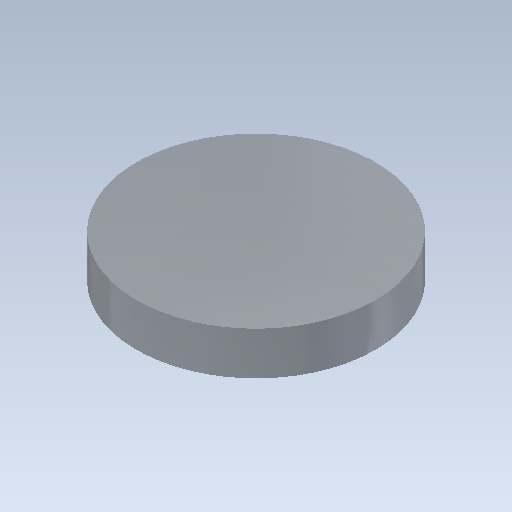
# Autodesk Inventor part: Borosilikatglas 55x10
Saved by Autodesk Inventor 2020.2 (Build 242310000, 310)
## iProperties
Created: 2012-12-10
Part Number: Borosilikatglas 55x10
Material: Glas
Document SubType Name: Modeling
Designer: g.schardt
Mass: 43.6646 g
Surface Area: 55.9243 cm^2
Volume: 20.0296 cm^3
Density: 2.18 g/cm^3
Appearance: Hellgrau
Project: 10W LED Lampenkopf
Author: g.schardt
Autodesk Inventor part; units mm, degrees
ref_plane "YZ Plane" through (0, 0, 0) normal (1, 0, 0) x (0, 1, 0)
ref_plane "XZ Plane" through (0, 0, 0) normal (0, 1, 0) x (-1, 0, 0)
ref_plane "XY Plane" through (0, 0, 0) normal (0, 0, 1) x (1, 0, 0)
sketch "Skizze1" plane through (0, 0, 0) normal (0, 0, 1) x (1, 0, 0)
  circle A0 centre (0, 0) radius 27.75
  dimension "d2" = 55.5
  constraints: 1 centre point
  measures "d2" diameter of A0
extrude "Extrusion1" add sketch "Skizze1" along normal blind 10
